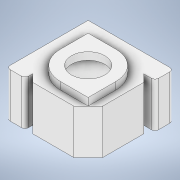
# Autodesk Inventor part: xy-mount-top
Saved by Autodesk Inventor 2020.4 (Build 244396000, 396)
## iProperties
Created: 2021-03-01
Part Number: xy-mount-top
Material: ABS Plastic
Document SubType Name: Modeling
Designer: AOB
Mass: 2.97661 g
Surface Area: 27.4332 cm^2
Volume: 2.80812 cm^3
Density: 1.06 g/cm^3
Appearance: Dark Green
Author: AOB
Autodesk Inventor part; units mm, degrees
ref_plane "YZ Plane" through (0, 0, 0) normal (1, 0, 0) x (0, 1, 0)
ref_plane "XZ Plane" through (0, 0, 0) normal (0, 1, 0) x (-1, 0, 0)
sketch "Sketch1" plane through (0, 0, 0) normal (0, 0, 1) x (1, 0, 0)
  line L0 (0, 0) -> (23, 0)
  line L1 (23, 0) -> (23, -24)
  line L2 (23, -24) -> (0, -24)
  line L3 (0, -24) -> (0, 0)
  line L4 (5, 0) -> (5, -24)
  line L5 (0, -24) -> (23, 0) construction
  line L6 (0, 0) -> (11.5, -12) construction
  dimension "d0" = 5
  dimension "d2" = 18
  dimension "d61" = 24
  constraints: 14 end point, 2 midpoint, 2 parallel, 2 perpendicular, 2 point on line, 1 horizontal
  measures "d0" distance of L0.start L4.start
  measures "d2" distance of L0.end L4.start
  measures "d61" distance of L0.end L1.end
extrude "Extrusion1" add sketch "Sketch1" along normal blind 17 contours L0 L4 L2 L3
extrude "Extrusion2" add sketch "Sketch1" against normal blind 5
sketch "Sketch2" plane through (0, 0, 0) normal (0, 0, 1) x (1, 0, 0)
  point P0 (0, 0)
  point P1 (11.0344, -10.0001)
hole "Hole1" at (11.0344, -10.0001, 0) direction (0, 0, -1) diameter 16 end through all
sketch "Sketch3" plane through (5, -24, 17) normal (1, 0, 0) x (0, 0, -1)
  line L0 (11.8812, 10.4951) -> (9.8812, 10.4951)
  point P0 (17, 24)
  constraints: 2 coincident, 2 end point, 4 other
hole "Hole2" at (5, -13.5049, 7.1188) direction (-1, 0, 0) diameter 16 end through all
fillet "Fillet2" radius 1 4 edges at (5, -12, 17) (0, -12, 17) (23, -12, 0) (23, -12, -5)
fillet "Fillet3" radius 0.1 3 edges at (5, -2.3739, 0) (5, -20.5775, 0) (5, -16.2036, 0)
sketch "Sketch5" plane through (0, 0, -5) normal (0, 1, 0) x (1, 0, 0)
  line L0 (5, -5) -> (5, -20.1188) projected
  line L1 (22, -5) -> (5.1, -5) construction
  line L2 (12.5, -5) -> (12.5, -12.5) construction
  line L3 (12.5, -12.5) -> (5, -12.5) construction
  circle A0 centre (12.5, -12.5) radius 7.5
  line L4 (12.5, -12.5) -> (16.8301, -5) construction
  line L5 (20, -12.5) -> (20.6263, -12.5) construction
  line L6 (16.8301, -5) -> (12.5, -5)
  line L7 (12.5, -12.5) -> (8.1699, -5) construction
  line L8 (8.1699, -5) -> (6.0048, -8.75)
  line L9 (12.5, -12.5) -> (3.8397, -12.5) construction
  line L10 (3.8397, -12.5) -> (6.0048, -16.25)
  line L11 (12.5, -12.5) -> (8.1699, -20)
  line L12 (8.1699, -20) -> (12.5, -20)
  line L13 (12.5, -12.5) -> (16.8301, -20) construction
  line L14 (16.8301, -20) -> (18.9952, -16.25)
  line L15 (12.5, -12.5) -> (21.1603, -12.5) construction
  line L16 (21.1603, -12.5) -> (18.9952, -8.75)
  line L17 (21.1603, -12.5) -> (18.9952, -16.25)
  line L18 (16.8301, -5) -> (18.9952, -8.75)
  line L19 (12.5, -5) -> (8.1699, -5)
  line L20 (3.8397, -12.5) -> (6.0048, -8.75)
  line L21 (8.1699, -20) -> (6.0048, -16.25)
  line L22 (16.8301, -20) -> (12.5, -20)
  point P0 (0, -5)
  point P1 (4.1, -4)
  point P2 (4, -4)
  point P3 (5.1, -5)
  point P4 (21, -4)
  dimension "d26" = 7.5
  dimension "d27" = 7.5
  dimension "d28" = 60
  dimension "d31" = 360
  constraints: 42 end point, 2 perpendicular, 2 point on circle, 2 tangent, 1 centre point, 1 coincident, 1 horizontal, 1 parallel, 1 point on line, 1 vertical, 35 other
  measures "d26" distance of L2.start L2.end
  measures "d27" distance of L2.end L3.end
  measures "d28" angle of L5 L4
ref_plane "Work Plane1" through (0, -12, -5) normal (0, 1, 0) x (1, 0, 0)
sketch "Sketch6" plane through (0, -12, -5) normal (0, 1, 0) x (1, 0, 0)
  circle A0 centre (12.5, -12.5) radius 7.5 projected
  line L0 (11.5, -19.933) -> (11.5, -21.933) construction
  line L1 (0, -21) -> (0, 0) projected
  line L2 (0, -25) -> (0, 0) construction
  line L3 (21.9591, -21.933) -> (7, -21.933)
  line L4 (21.9591, -7) -> (21.9591, -21.933)
  line L5 (5, -5.1) -> (5, -19.933)
  line L6 (19.9591, -13.2818) -> (21.9591, -13.2818) construction
  line L7 (11.5, -19.933) -> (11.5, -21.933) construction
  line L8 (1, -22) -> (4, -22) projected
  line L9 (5, -5) -> (5, -20.1188) projected
  line L10 (18.681, -8.252) -> (20.0952, -6.8378)
  line L11 (19.0344, -5) -> (5.1, -5) projected
  line L12 (7.6058, -18.183) -> (6.1916, -19.5972) construction
  line L13 (6.1916, -19.5972) -> (5, -18.4057)
  spline S0 degree 2 poles (5.1, -5) (5, -5) (5, -5.1) knots 0 0 0 1 1 1 weights 1 0.707107 1 projected
  line L14 (7, -21.933) -> (5, -19.933)
  line L15 (5.1, -5) -> (19.9591, -5)
  line L16 (21.9591, -7) -> (19.9591, -5)
  point P0 (0, -5)
  point P1 (21.9591, -5)
  point P2 (21.9591, -8.7017)
  point P3 (5, -5)
  point P4 (5, -19.933)
  point P5 (8.5274, -21.933)
  point P6 (18.2574, -5)
  point P7 (12.5, -5)
  point P8 (5, -12.5)
  point P9 (5, -21.933)
  point P10 (21.9591, -5)
  point P11 (12.5, -5)
  dimension "d94" = 2
  dimension "d95" = 2
  dimension "d98" = 2
  dimension "d99" = 2
  dimension "d100" = 2
  dimension "d101" = 2
  dimension "d102" = 2
  dimension "d103" = 2
  constraints: 26 end point, 14 point on line, 4 point on circle, 2 vertical, 1 collinear, 1 horizontal, 1 perpendicular, 2 other
  measures "d94" distance of L0.start L7.end
  measures "d95" distance of L6.start L6.end
  measures "d98" distance of L10.start L10.end
  measures "d99" distance of L12.start L12.end
  measures "d100" distance of L3.end point (5, -21.933)
  measures "d101" distance of L5.end point (5, -21.933)
  measures "d102" distance of L4.start point (21.959, -5)
  measures "d103" distance of L15.end point (21.959, -5)
extrude "Extrusion3" add sketch "Sketch6" along normal mid plane 24 contours A0 L11 L15 L16 L4 L3 L14 L5 | L5 S0 L11 A0
sketch "Sketch7" plane through (0, 0, -5) normal (0, 1, 0) x (1, 0, 0)
  circle A0 centre (12.5, -12.5) radius 7.5
  circle A1 centre (12.5, -12.5) radius 4.5
  circle A2 centre (12.5, -12.5) radius 7.5 projected
  line L0 (19.9591, -5) -> (22, -5) projected
  line L1 (5, -20) -> (20, -20)
  line L2 (20, -20) -> (20, -5)
  line L3 (20, -5) -> (5, -5)
  line L4 (5, -5) -> (5, -20)
  point P0 (5, -12.5)
  point P1 (12.5, -5)
  point P2 (20, -12.5)
  point P3 (12.5, -20)
  dimension "d82" = 9
  constraints: 8 end point, 2 centre point, 2 coincident, 2 parallel, 1 horizontal, 1 perpendicular, 1 point on line
  measures "d82" diameter of A1
extrude "Extrusion4" add sketch "Sketch7" along normal blind 2 contours A0 | L2 L1 A0 | A0 L4 L3
mirror "Mirror1" about plane through (0, -12, -5) normal (0, 1, 0) of "Extrusion4"
chamfer "Chamfer2" distance 3.9 angle 45 1 edges at (21.9591, -12, 16.933)
split "Split2" plane through (0, -12, -5) removes the side toward (0, -1, 0)
body "Solid1"
